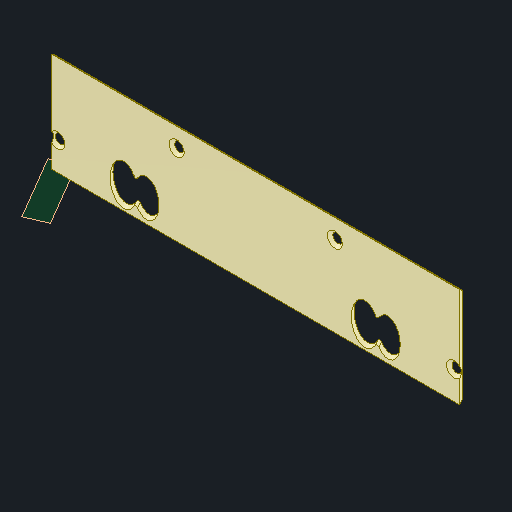
# Autodesk Inventor part: front
Saved by Autodesk Inventor 2023 (Build 270158000, 158)
## iProperties
Created: 2024-05-20
Part Number: front
Material: Nylon 6/6
Document SubType Name: Modeling
Designer: szymo
Density: 1.13 g/cm^3
Appearance: Nylon 6
Mass: 9.2658 g
Surface Area: 147.118 cm^2
Volume: 8.19983 cm^3
Author: szymo
Autodesk Inventor part; units mm, degrees
ref_plane "YZ Plane" through (0, 0, 0) normal (1, 0, 0) x (0, 1, 0)
ref_plane "XZ Plane" through (0, 0, 0) normal (0, 1, 0) x (-1, 0, 0)
ref_plane "Work Plane1" through (0, -45.8455, -0.8595) normal (-1, 0, 0) x (0, 0.5735764, 0.819152)
sketch "Sketch1" plane through (0, -45.8455, -0.8595) normal (-1, 0, 0) x (0, 0.5735764, 0.819152)
  line L0 (4.2002, 4.5) -> (27, 37.0615) projected
  line L1 (3.5, -0.5) -> (3.5, 3.5) projected
  line L2 (27, 37.0615) -> (28, 37.0615) projected
  line L3 (27, 37.0615) -> (3.5, 3.5)
  line L4 (3.5, 1.4079) -> (28.4649, 37.0615)
  line L5 (27, 37.0615) -> (28.4649, 37.0615)
  point P0 (4.2002, 4.5)
  dimension "d0" = 1.2
  dimension "d1" = 55
  constraints: 6 end point, 1 collinear, 1 parallel, 1 point on line
  measures "d0" distance between parallel lines of L3 L4
  measures "d1" angle of L4 L5
ref_plane "Work Plane2" through (178, -42.7329, -77.104) normal (1, 0, 0) x (0, 0.819152, -0.5735764)
extrude "Extrusion1" add sketch "Sketch1" against normal up to surface (178 mm away)
ref_plane "Work Plane3" through (36.3849, -23.4357, -7.1547) normal (0, -0.7489557, 0.66262) x (1, 0, 0)
ref_plane "Work Plane4" through (36.3849, -23.4357, -7.1547) normal (0, -0.7489557, 0.66262) x (1, 0, 0)
sketch "Sketch4" plane through (36.3849, -23.4357, -7.1547) normal (0, -0.7489557, 0.66262) x (1, 0, 0)
  line L0 (-14.9215, 5.4518) -> (-14.9215, -5.4534)
  spline S0 degree 3 poles (-14.9215, -5.4534) (-14.9222, -5.5772) (-14.8715, -5.6989) (-14.7851, -5.7853) (-14.7653, -5.8051) (-14.7437, -5.823) (-14.7206, -5.8388) (-14.7012, -5.8521) (-14.6808, -5.864) (-14.6595, -5.8743) (-14.6436, -5.882) (-14.6272, -5.8889) (-14.6105, -5.8948) (-14.5603, -5.9125) (-14.5071, -5.9218) (-14.4534, -5.9215) knots 0 0 0 0 0.5 0.5 0.5 0.614375 0.614375 0.614375 0.710781 0.710781 0.710781 0.783086 0.783086 0.783086 1 1 1 1
  line L1 (-14.4534, -5.9215) -> (14.4534, -5.9215)
  spline S1 degree 3 poles (14.4534, -5.9215) (14.5775, -5.9222) (14.6994, -5.8713) (14.8723, -5.6977) (14.9222, -5.5758) (14.9215, -5.4518) knots 0 0 0 0 0.5 0.5 1 1 1 1
  line L2 (14.9215, -5.4518) -> (14.9215, 5.4534)
  spline S2 degree 3 poles (14.9215, 5.4534) (14.9222, 5.5775) (14.8713, 5.6994) (14.6977, 5.8723) (14.5758, 5.9222) (14.4518, 5.9215) knots 0 0 0 0 0.5 0.5 1 1 1 1
  line L3 (14.4518, 5.9215) -> (-14.4534, 5.9215)
  spline S3 degree 3 poles (-14.4534, 5.9215) (-14.5775, 5.9222) (-14.6994, 5.8713) (-14.8723, 5.6977) (-14.9222, 5.5758) (-14.9215, 5.4518) knots 0 0 0 0 0.5 0.5 1 1 1 1
  circle A0 centre (-13.3791, -4.3791) radius 0.5
  circle A1 centre (-13.3791, 4.3791) radius 0.5
  circle A2 centre (13.3791, 4.3791) radius 0.5
  circle A3 centre (13.3791, -4.3791) radius 0.5
  arc A4 (0.2617, -1.4512) -> (0.1811, -1.5218) centre (0.2771, -1.55) ccw
  arc A5 (0.1811, 1.5218) -> (0.1811, -1.5218) centre (-5, 0) ccw
  arc A6 (0.1811, 1.5218) -> (0.2617, 1.4512) centre (0.2771, 1.55) ccw
  arc A7 (0.2617, 1.4512) -> (0.3414, 1.519) centre (0.2463, 1.55) ccw
  arc A8 (0.3414, -1.519) -> (0.3414, 1.519) centre (5, 0) ccw
  arc A9 (0.3414, -1.519) -> (0.2617, -1.4512) centre (0.2463, -1.55) ccw
  line L4 (90.3087, 5.4518) -> (90.3087, -5.4534)
  spline S4 degree 3 poles (90.3087, -5.4534) (90.308, -5.5772) (90.3587, -5.6989) (90.4451, -5.7853) (90.4649, -5.8051) (90.4865, -5.823) (90.5096, -5.8388) (90.529, -5.8521) (90.5494, -5.864) (90.5707, -5.8743) (90.5866, -5.882) (90.603, -5.8889) (90.6197, -5.8948) (90.6699, -5.9125) (90.7231, -5.9218) (90.7769, -5.9215) knots 0 0 0 0 0.5 0.5 0.5 0.614375 0.614375 0.614375 0.710781 0.710781 0.710781 0.783086 0.783086 0.783086 1 1 1 1
  line L5 (90.7769, -5.9215) -> (119.6836, -5.9215)
  spline S5 degree 3 poles (119.6836, -5.9215) (119.8077, -5.9222) (119.9296, -5.8713) (120.1025, -5.6977) (120.1524, -5.5758) (120.1517, -5.4518) knots 0 0 0 0 0.5 0.5 1 1 1 1
  line L6 (120.1517, -5.4518) -> (120.1517, 5.4534)
  spline S6 degree 3 poles (120.1517, 5.4534) (120.1524, 5.5775) (120.1015, 5.6994) (119.9279, 5.8723) (119.806, 5.9222) (119.682, 5.9215) knots 0 0 0 0 0.5 0.5 1 1 1 1
  line L7 (119.682, 5.9215) -> (90.7769, 5.9215)
  spline S7 degree 3 poles (90.7769, 5.9215) (90.6527, 5.9222) (90.5308, 5.8713) (90.3579, 5.6977) (90.308, 5.5758) (90.3087, 5.4518) knots 0 0 0 0 0.5 0.5 1 1 1 1
  circle A10 centre (91.8511, -4.3791) radius 0.5
  circle A11 centre (91.8511, 4.3791) radius 0.5
  circle A12 centre (118.6093, 4.3791) radius 0.5
  circle A13 centre (118.6093, -4.3791) radius 0.5
  arc A14 (105.4919, -1.4512) -> (105.4113, -1.5218) centre (105.5073, -1.55) ccw
  arc A15 (105.4113, 1.5218) -> (105.4113, -1.5218) centre (100.2302, 0) ccw
  arc A16 (105.4113, 1.5218) -> (105.4919, 1.4512) centre (105.5073, 1.55) ccw
  arc A17 (105.4919, 1.4512) -> (105.5716, 1.519) centre (105.4765, 1.55) ccw
  arc A18 (105.5716, -1.519) -> (105.5716, 1.519) centre (110.2302, 0) ccw
  arc A19 (105.5716, -1.519) -> (105.4919, -1.4512) centre (105.4765, -1.55) ccw
  arc A20 (105.5127, 2.6278) -> (105.5127, -2.6278) centre (100.2302, 0) ccw
  arc A21 (105.5127, -2.6278) -> (105.5127, 2.6278) centre (110.2302, 0) ccw
  arc A22 (0.2825, 2.6278) -> (0.2825, -2.6278) centre (-5, 0) ccw
  arc A23 (0.2825, -2.6278) -> (0.2825, 2.6278) centre (5, 0) ccw
  point P0 (-36.3849, 20.8875)
  dimension "d27" = 0.5
  dimension "d28" = 0.5
  constraints: 8 point on circle, 4 centre point, 2 other
  measures "d27" radial gap between concentric circles of A18 A21
  measures "d28" radial gap between concentric circles of A8 A23
extrude "Extrusion2" cut sketch "Sketch4" along normal up to next contours A4 A5 A6 A7 A8 A9 | A14 A15 A16 A17 A18 A19 | A21 A20 | A23 A22
sketch "Sketch6" plane through (0, -42.6848, 1.2) normal (0, 0, 1) x (1, 0, 0)
  circle A0 centre (54.5, 35.1848) radius 2.3 projected
  circle A1 centre (123.5, 35.1848) radius 2.3 projected
  circle A2 centre (2.5, 12.2262) radius 2.3 projected
  circle A3 centre (175.5, 12.2262) radius 2.3 projected
  point P0 (0, 42.6848)
  constraints: 4 coincident
hole "Hole1" at (54.5, -7.5, 1.2) at (123.5, -7.5, 1.2) at (2.5, -30.4585, 1.2) at (175.5, -30.4585, 1.2) direction (0, 0, -1) diameter 3.6 end through all countersink diameter 6.6 countersink angle 90 clearance for "Countersunk Flat Head Screw ISO 2009/7046" size "M3" standard "ISO"
fillet "Fillet1" radius 1 4 edges at (36.6674, -36.1666, 0.6) (36.6674, -28.2351, 0.6) (141.8976, -28.2351, 0.6) (141.8976, -36.1666, 0.6)
body "Solid1"
